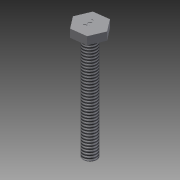
# Autodesk Inventor part: .25 diameter 2'' bolt
Saved by Autodesk Inventor 2011 SP1 (Build 150282100, 282)
## iProperties
Created: 2013-01-18
Part Number: .25 diameter 2'' bolt
Document SubType Name: Modeling
Designer: wes
Density: 1 g/cm^3
Author: wes
Autodesk Inventor part; units mm, degrees
ref_plane "YZ Plane" through (0, 0, 0) normal (1, 0, 0) x (0, 1, 0)
ref_plane "XZ Plane" through (0, 0, 0) normal (0, 1, 0) x (-1, 0, 0)
ref_plane "XY Plane" through (0, 0, 0) normal (0, 0, 1) x (1, 0, 0)
sketch "Sketch1" plane through (0, 0, 0) normal (0, 0, 1) x (1, 0, 0)
  line L0 (-17.9641, 33.2251) -> (-14.7891, 33.2251)
  line L1 (-14.7891, 33.2251) -> (-14.7891, -17.5749)
  line L2 (-14.7891, -17.5749) -> (-17.9641, -17.5749)
  line L3 (-17.9641, -17.5749) -> (-17.9641, 33.2251)
  point P0 (0, 0)
  dimension "d0" = 3.175
  dimension "d1" = 50.8
  constraints: 8 end point, 2 parallel, 1 horizontal, 1 perpendicular
  measures "d0" distance of L1.end L2.end
  measures "d1" distance of L0.end L1.end
revolve "Revolution1" add sketch "Sketch1" angle 360 about axis through (-17.9641, -17.5749, 0) along (0, 1, 0)
sketch "Sketch2" plane through (-17.9641, 33.2251, 0) normal (0, 1, 0) x (1, 0, 0)
  circle A0 centre (0, 0) radius 3.175 projected
  line L0 (-2.7933, -6.7141) -> (-7.2112, -0.938)
  line L1 (-7.2112, -0.938) -> (-4.418, 5.7761)
  line L2 (-4.418, 5.7761) -> (2.7933, 6.7141)
  line L3 (2.7933, 6.7141) -> (7.2112, 0.938)
  line L4 (7.2112, 0.938) -> (4.418, -5.7761)
  line L5 (4.418, -5.7761) -> (-2.7933, -6.7141)
  point P0 (17.9641, 0)
  constraints: 12 end point, 1 coincident, 13 other
extrude "Extrusion1" add sketch "Sketch2" along normal blind 3.81 contours A0 | L0 L1 L2 L3 L4 L5
thread "Thread1" size "1/4-20 UNC" class "2A" standard "ANSI Unified Screw Threads" full length
sketch "Sketch3" plane through (-17.9641, 37.0351, 0) normal (0, 1, 0) x (1, 0, 0)
  spline S0 degree 5 poles (-1.6705, -1.7697) (-1.5087, -1.85) (-0.562, -1.832) (2.4108, -1.3359) (-1.0538, -0.5942) (-0.3082, 0.5963) (2.0933, -0.7076) (-1.4851, 3.8244) (-2.0876, 1.526) (-0.2865, 2.0954) (0.0858, 0.4541) (-1.2327, 0.9989) (-1.1868, -0.5585) (0.1138, -0.9114) (-0.367, -1.1465) (-1.6028, -1.5407) (-1.7853, -1.7128) (-1.6705, -1.7697) knots 0 0 0 0 0 0 0.118263 0.184405 0.277398 0.35545 0.432093 0.511849 0.589546 0.655005 0.725096 0.791185 0.859928 0.916088 1 1 1 1 1 1
  point P0 (17.9641, 0)
  point P1 (-0.2467, -0.2687)
  point P2 (-0.1215, 0.0477)
  point P3 (0.7392, 0.3)
  point P4 (-1.3859, 2.4418)
  point P5 (-1.4827, 2.0902)
  point P6 (-0.4576, 1.5038)
  point P7 (-0.3161, 0.9046)
  point P8 (-0.8855, 0.5658)
  point P9 (-0.8855, -0.3278)
  point P10 (-0.3187, -0.9153)
  point P11 (-0.8855, -1.3006)
  constraints: 13 other
extrude "Extrusion2" cut sketch "Sketch3" against normal blind 0.254
body "Solid1"
